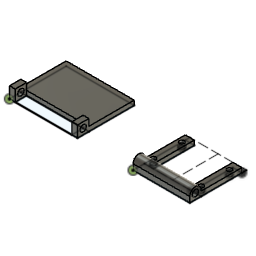
raspi_camera v3 (Autodesk Fusion 360 design; units mm, degrees)
Autodesk Fusion 360 part; units mm, degrees
sketch "スケッチ1" plane through (0, 0, 0) normal (0, 0, 1) x (1, 0, 0)
  line L0 (15.4645, 12.5405) -> (45.4645, 12.5405) construction
  line L1 (45.4645, 12.5405) -> (45.4645, 32.5405)
  line L2 (45.4645, 32.5405) -> (15.4645, 32.5405)
  line L3 (15.4645, 32.5405) -> (15.4645, 12.5405)
  line L4 (70, 12.5405) -> (95, 12.5405) construction
  line L5 (95, 12.5405) -> (95, 32.5405)
  line L6 (95, 32.5405) -> (70, 32.5405) construction
  line L7 (70, 32.5405) -> (70, 12.5405)
  line L8 (72, 32.5405) -> (72, 12.5405) construction
  circle A0 centre (72, 27.0405) radius 1.05
  circle A1 centre (72, 14.5405) radius 1.05
  line L9 (82.5, 32.5405) -> (82.5, 12.5405) construction
  circle A2 centre (93, 27.0405) radius 1.05
  circle A3 centre (93, 14.5405) radius 1.05
  line L10 (70, 30.5405) -> (74, 30.5405)
  line L11 (74, 30.5405) -> (74, 12.5405)
  line L12 (91, 30.5405) -> (91, 12.5405)
  line L13 (95, 30.5405) -> (91, 30.5405)
  line L14 (70, 12.5405) -> (95, 12.5405)
  line L15 (95, 12.5405) -> (95, 7.5405)
  line L16 (95, 7.5405) -> (70, 7.5405)
  line L17 (70, 7.5405) -> (70, 12.5405)
  line L18 (15.4645, 12.5405) -> (45.4645, 12.5405)
  line L19 (45.4645, 12.5405) -> (45.4645, 7.5405)
  line L20 (45.4645, 7.5405) -> (15.4645, 7.5405)
  line L21 (15.4645, 7.5405) -> (15.4645, 12.5405)
  line L22 (17.9645, 12.5405) -> (42.9645, 12.5405)
  line L23 (42.9645, 12.5405) -> (42.9645, 7.5405)
  line L24 (42.9645, 7.5405) -> (17.9645, 7.5405)
  line L25 (17.9645, 7.5405) -> (17.9645, 12.5405)
  dimension "d1" = 30
  dimension "d2" = 20
  dimension "d3" = 25
  dimension "d4" = 20
  dimension "d5" = 2
  dimension "d7" = 2.1
  dimension "d8" = 2.1
  dimension "d11" = 12.5
  dimension "d12" = 2
  dimension "d13" = 4
  dimension "d14" = 18
  dimension "d15" = 25
  dimension "d16" = 5
  dimension "d18" = 5
  dimension "d19" = 25
  dimension "d20" = 5
  dimension "d21" = 2.5
  constraint horizontal L0
  constraint vertical L1
  constraint horizontal L2
  constraint vertical L3
  constraint horizontal L4
  constraint vertical L5
  constraint horizontal L6
  constraint vertical L7
  constraint collinear L0 L4
  constraint coincident L6 L8.start
  constraint coincident L4 L8.end
  constraint perpendicular L4 L8
  constraint coincident L8 A0.centre
  constraint coincident L8 A1.centre
  constraint midpoint L6 L9.start
  constraint midpoint L4 L9.end
  constraint symmetric A0 L9 A2
  constraint symmetric A1 L9 A3
  constraint coincident L7 L10.start
  constraint perpendicular L8 L10
  constraint coincident L4 L11.end
  constraint perpendicular L4 L11
  constraint symmetric L9 L10.start L13.start
  constraint symmetric L9 L10.end L12.start
  constraint symmetric L9 L11.end L12.end
  constraint horizontal L14
  constraint vertical L15
  constraint horizontal L16
  constraint vertical L17
  constraint horizontal L18
  constraint vertical L19
  constraint horizontal L20
  constraint vertical L21
  constraint collinear L1 L19
  constraint horizontal L22
  constraint vertical L23
  constraint horizontal L24
  constraint vertical L25
  constraint coincident L18 L22.start
  measures "d1" distance of L0.start L0.end
  measures "d2" distance of L0.start L2.end
  measures "d3" distance of L4.start L4.end
  measures "d4" distance of L4.start L6.end
  measures "d5" distance of L7 L8
  measures "d7" diameter of A0
  measures "d8" diameter of A1
  measures "d11" distance of A0.centre A1.centre
  measures "d12" distance of L4 A1.centre
  measures "d13" distance of L10.start L10.end
  measures "d14" distance of L4.start L10.start
  measures "d15" distance of L4.start L4.end
  measures "d16" distance of L4.start L16.end
  measures "d18" distance of L0.start L20.end
  measures "d19" distance of L22.start L22.end
  measures "d20" distance of L22.start L24.end
  measures "d21" distance of L21 L25
extrude "押し出し1" add sketch "スケッチ1" along normal blind 2 contours L1 L2 L3 L18 L22 makes body 1
extrude "押し出し2" add sketch "スケッチ1" along normal blind 2 separate body contours L5 L12 L13 L14 | L7 L10 L11 L14 makes body 2 at (72.0262, 29.7228, 0) makes body 3 at (92.9738, 29.7228, 0)
extrude "押し出し3" add sketch "スケッチ1" along normal blind 5 contours L18 L19 L20 L23 | L18 L20 L21 L25 bodies 1
extrude "押し出し4" add sketch "スケッチ1" along normal blind 5 contours L14 L15 L16 L17 bodies 2 3
sketch "スケッチ2" plane through (15.4645, 0, 0) normal (-1, 0, 0) x (0, -1, 0)
  line L0 (-32.5405, 0) -> (-7.5405, 0)
  line L1 (-7.5405, 0) -> (-7.5405, 5)
  line L2 (-7.5405, 5) -> (-12.5405, 5)
  line L3 (-12.5405, 5) -> (-12.5405, 2)
  line L4 (-12.5405, 2) -> (-32.5405, 2)
  line L5 (-32.5405, 2) -> (-32.5405, 0)
  circle A0 centre (-10.0405, 2.5) radius 1.4
  dimension "d30" = 2.8
  dimension "d31" = 2.5
  dimension "d32" = 2.5
  measures "d30" diameter of A0
  measures "d31" distance of L1 A0.centre
  measures "d32" distance of L2 A0.centre
extrude "押し出し5" cut sketch "スケッチ2" against normal blind 99 contours A0 bodies 1 2
fillet "フィレット1" radius 2.5 2 edges at (82.5, 7.5405, 5) (82.5, 12.5405, 5) on bodies 2
